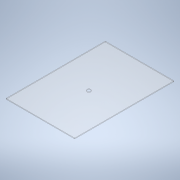
# Autodesk Inventor part: newbottom
Saved by Autodesk Inventor 2020.1 (Build 241239000, 239)
## iProperties
Created: 2021-08-04
Part Number: newbottom
Material: PMMA Plastic
Document SubType Name: Modeling
Designer: Caleb
Density: 1.188 g/cm^3
Appearance: Polycarbonate - Clear
Author: Caleb
Autodesk Inventor part; units mm, degrees
ref_plane "YZ Plane" through (0, 0, 0) normal (1, 0, 0) x (0, 1, 0)
ref_plane "XZ Plane" through (0, 0, 0) normal (0, 1, 0) x (-1, 0, 0)
ref_plane "XY Plane" through (0, 0, 0) normal (0, 0, 1) x (1, 0, 0)
sketch "Sketch1" plane through (0, 0, 0) normal (0, 1, 0) x (-1, 0, 0)
  line L0 (225, 317.9348) -> (-225, 317.9348)
  line L1 (-225, 317.9348) -> (-225, -332.0652)
  line L2 (-225, -332.0652) -> (225, -332.0652)
  line L3 (225, -332.0652) -> (225, 317.9348)
  point P0 (0, 0)
  dimension "d11" = 450
  dimension "d12" = 650
  constraints: 8 end point, 2 parallel, 1 horizontal, 1 perpendicular
  measures "d11" distance between parallel lines of L1 L3
  measures "d12" distance of L2.end L0.start
extrude "Extrusion1" add sketch "Sketch1" along normal mid plane 5
sketch "Sketch2" plane through (0, 2.5, 0) normal (0, 1, 0) x (1, 0, 0)
  point P0 (0, 0)
hole "Hole1" at (0, 2.5, 0) direction (0, -1, 0) diameter 22.7 end through all
body "Solid1"
